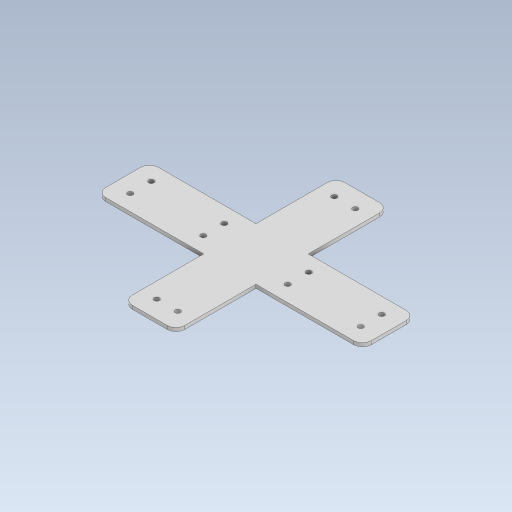
# Autodesk Inventor part: Konektor Casis
Saved by Autodesk Inventor 2023.5 (Build 275446000, 446)
## iProperties
Created: 2025-09-16
Part Number: Konektor Casis
Material: Generic
Document SubType Name: Modeling
Designer: Guntur
Density: 1 g/cm^3
Appearance: Default
Author: Guntur
## iProperties of the stored document Konektor Casis_3DPrint.ipt
Created: 2025-09-20
Part Number: Konektor Casis_3DPrint
Material: Generic
Document SubType Name: Modeling
Designer: Guntur
Density: 1 g/cm^3
Appearance: Default
Author: Guntur
Autodesk Inventor part; units mm, degrees
ref_plane "YZ Plane" through (0, 0, 0) normal (1, 0, 0) x (0, 1, 0)
ref_plane "XZ Plane" through (0, 0, 0) normal (0, 1, 0) x (-1, 0, 0)
ref_plane "XY Plane" through (0, 0, 0) normal (0, 0, 1) x (1, 0, 0)
sketch "Sketch1" plane through (0, 0, 0) normal (0, 1, 0) x (-1, 0, 0)
  line L0 (0, -273.05) -> (0, 296.8625) construction
  line L1 (373.0625, 0) -> (-258.7625, 0) construction
  circle A0 centre (24.125, -6) radius 1.5
  circle A1 centre (65.875, -6) radius 1.5
  circle A2 centre (24.125, 6) radius 1.5
  circle A3 centre (65.875, 6) radius 1.5
  circle A4 centre (-24.125, -6) radius 1.5
  circle A5 centre (-65.875, -6) radius 1.5
  circle A6 centre (-24.125, 6) radius 1.5
  circle A7 centre (-65.875, 6) radius 1.5
  circle A8 centre (6, 50.75) radius 1.5
  circle A9 centre (-6, 50.75) radius 1.5
  circle A10 centre (6, -50.75) radius 1.5
  circle A11 centre (-6, -50.75) radius 1.5
  line L2 (75.875, 0) -> (75.875, -10)
  line L3 (70.875, -15) -> (15, -15)
  line L4 (0, -60.75) -> (10, -60.75)
  line L5 (15, -55.75) -> (15, -15)
  arc A12 (70.875, -15) -> (75.875, -10) centre (70.875, -10) ccw
  arc A13 (10, -60.75) -> (15, -55.75) centre (10, -55.75) ccw
  line L6 (-75.875, 0) -> (-75.875, -10)
  line L7 (-70.875, -15) -> (-15, -15)
  line L8 (0, -60.75) -> (-10, -60.75)
  line L9 (-15, -55.75) -> (-15, -15)
  arc A14 (-15, -55.75) -> (-10, -60.75) centre (-10, -55.75) ccw
  arc A15 (-75.875, -10) -> (-70.875, -15) centre (-70.875, -10) ccw
  line L10 (75.875, 0) -> (75.875, 10)
  line L11 (70.875, 15) -> (15, 15)
  line L12 (0, 60.75) -> (10, 60.75)
  line L13 (15, 55.75) -> (15, 15)
  arc A16 (75.875, 10) -> (70.875, 15) centre (70.875, 10) ccw
  arc A17 (15, 55.75) -> (10, 60.75) centre (10, 55.75) ccw
  line L14 (-70.875, 15) -> (-15, 15)
  line L15 (-75.875, 0) -> (-75.875, 10)
  line L16 (-15, 55.75) -> (-15, 15)
  arc A18 (-10, 60.75) -> (-15, 55.75) centre (-10, 55.75) ccw
  line L17 (0, 60.75) -> (-10, 60.75)
  arc A19 (-70.875, 15) -> (-75.875, 10) centre (-70.875, 10) ccw
  point P0 (0, 0)
  point P1 (75.875, -15)
  point P2 (15, -60.75)
  point P3 (75.875, 15)
  point P4 (15, 60.75)
  dimension "d1" = 24.125
  dimension "d3" = 6
  dimension "d4" = 3
  dimension "d5" = 41.75
  dimension "d6" = 3
  dimension "d7" = 50.75
  dimension "d8" = 6
  dimension "d9" = 15
  dimension "d10" = 10
  dimension "d11" = 15
  dimension "d12" = 10
  dimension "d13" = 5
  dimension "d14" = 5
  constraints: 36 end point, 34 symmetric about line, 20 centre point, 16 point on circle, 10 point on line, 4 tangent, 3 horizontal, 3 vertical, 2 perpendicular, 16 other
  measures "d1" distance from line of L0 A0.centre
  measures "d3" distance from line of L1 A0.centre
  measures "d4" diameter of A1
  measures "d5" distance of A1.centre A0.centre
  measures "d6" diameter of A8
  measures "d7" distance from line of L1 A8.centre
  measures "d8" distance from line of L0 A8.centre
  measures "d9" distance of L2.start point (75.875, -15)
  measures "d10" distance from line of L2 A1.centre
  measures "d11" distance of L4.start point (15, -60.75)
  measures "d12" distance from line of L4 A10.centre
  measures "d13" radius of A12
  measures "d14" radius of A13
extrude "Extrusion1" add sketch "Sketch1" along normal blind 2
body "Solid1"
